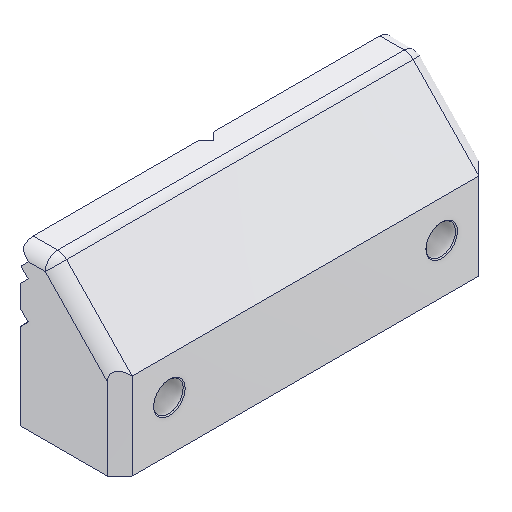
# Autodesk Inventor part: 3DP_ABS_Jaw_Second_Half
Saved by Autodesk Inventor 2026.1 (Build 301233000, 233)
## iProperties
Created: 2018-02-17
Part Number: 3DP_ABS_Jaw_Second_Half
Material: Ogólny
Document SubType Name: Modeling
Designer: Andrzej
Density: 1 g/cm^3
Appearance: PTFE
Mass: 38.2435 g
Surface Area: 91.1302 cm^2
Volume: 38.2435 cm^3
Author: Andrzej
Autodesk Inventor part; units mm, degrees
ref_plane "YZ Plane" through (0, 0, 0) normal (1, 0, 0) x (0, 1, 0)
ref_plane "XZ Plane" through (0, 0, 0) normal (0, 1, 0) x (-1, 0, 0)
sketch "Szkic1" plane through (0, 0, 0) normal (0, 0, 1) x (1, 0, 0)
  line L0 (-10, 37.5) -> (10, 37.5)
  line L1 (10, 37.5) -> (10, -37.5)
  line L2 (10, -37.5) -> (-10, -37.5)
  line L3 (-10, -37.5) -> (-10, 37.5)
  point P0 (0, 0)
  dimension "d0" = 20
  dimension "d1" = 75
  dimension "d39" = 37.5
  dimension "d40" = 10
  constraints: 8 end point, 2 parallel, 1 horizontal, 1 perpendicular
  measures "d0" distance of L1.end L2.end
  measures "d1" distance of L0.end L1.end
  measures "d39" distance from line of point (0, 0) L0
  measures "d40" distance from line of point (0, 0) L1
extrude "Wyciągnięcie proste1" add sketch "Szkic1" along normal blind 32
sketch "Szkic2" plane through (10, -37.5, 0) normal (1, 0, 0) x (0, 0, -1)
  line L0 (0, 75) -> (0, 0) projected
  line L1 (0, 75) -> (-32, 75) projected
  line L2 (-32, 0) -> (-32, 75) projected
  line L3 (0, 0) -> (-32, 0) projected
  point P0 (0, 37.5)
  point P1 (-10, 10)
  point P2 (-10, 65)
  dimension "d4" = 32
  dimension "d5" = 10
  dimension "d6" = 10
  dimension "d7" = 10
  dimension "d8" = 10
  measures "d4" distance of L0.end L2.start
  measures "d5" distance from line of L0 point (-10, 10)
  measures "d6" distance from line of L0 point (-10, 65)
  measures "d7" distance from line of L3 point (-10, 10)
  measures "d8" distance from line of L1 point (-10, 65)
hole "Otwór1" at (10, -27.5, 10) at (10, 27.5, 10) direction (-1, 0, 0) diameter 6 end through all
sketch "Szkic3" plane through (-10, 37.5, 0) normal (0, 1, 0) x (1, 0, 0)
  line L0 (0, 0) -> (20, 0) projected
  line L1 (0, 0) -> (0, -32) projected
  line L2 (20, -32) -> (0, -32) projected
  line L3 (20, 0) -> (20, -32) projected
  line L4 (0, -28) -> (1.5, -26.5)
  line L5 (0, -28) -> (2.2095, -28) construction
  line L6 (0, 0) -> (0, -32) projected
  line L7 (0, -25) -> (1.5, -26.5)
  line L8 (0, -25) -> (2.7592, -25) construction
  dimension "d17" = 45
  dimension "d19" = 45
  dimension "d20" = 3
  dimension "d21" = 4
  constraints: 8 end point, 2 horizontal, 2 point on line
  measures "d17" angle of L5 L4
  measures "d19" angle of L7 L8
  measures "d20" distance of L7.start L4.start
  measures "d21" distance from line of L2 L4.start
extrude "Wyciągnięcie proste2" cut sketch "Szkic3" against normal through all contours L7 L4 L1
chamfer "Faza1" distance 14 distance2 14.5 1 edges at (10, 0, 32) measured on face at (-3.3333, 12.5, 32)
chamfer "Faza2" distance 2.5 angle 45 2 edges at (10, -37.5, 8.75) (10, 37.5, 8.75)
ref_plane "Płaszczyzna konstrukcyjna1" through (-10, 37.5, 32) normal (0, -0.9902681, -0.1391731) x (-1, 0, 0)
sketch "Szkic4" plane through (-10, 37.5, 32) normal (0, -0.9902681, -0.1391731) x (-1, 0, 0)
  line L0 (-17.5, 31.6886) -> (-17.5, 11.7948) projected
  line L1 (0, 31.6886) -> (-17.5, 31.6886) projected
  line L2 (0, 31.6886) -> (0, 6.9319) projected
  line L3 (0, 6.9319) -> (-1.5, 5.4465) projected
  line L4 (-1.5, 5.4465) -> (0, 3.9611) projected
  line L5 (0, 3.9611) -> (0, 0) projected
  line L6 (-6, 0) -> (0, 0) projected
  line L7 (-17.5, 11.7948) -> (-6, 0) projected
  line L8 (0, -3.5061) -> (0, 6.9319) projected
  line L9 (0, 1) -> (-1.5, 2.5)
  line L10 (0, 1) -> (2.5951, 1) construction
  line L11 (0, 31.6886) -> (0, 6.9319) projected
  line L12 (0, 4) -> (-1.5, 2.5)
  line L13 (0, 4) -> (3.5979, 4) construction
  line L14 (0, 1) -> (0, 4)
  point P0 (-10, 26.4696)
  dimension "d32" = 135
  dimension "d34" = 135
  dimension "d35" = 3
  dimension "d36" = 1
  constraints: 10 end point, 2 horizontal, 2 point on line, 1 collinear
  measures "d32" angle of L10 L9
  measures "d34" angle of L12 L13
  measures "d35" distance of L12.start L9.start
  measures "d36" distance of L5.end L9.start
extrude "Wyciągnięcie proste3" cut sketch "Szkic4" along normal through all contours L8 L4 L12 | L9 L12 L4 L5
mirror "Odbicie lustrzane1" about plane through (0, 0, 0) normal (0, 1, 0) of "Wyciągnięcie proste3"
sketch "Szkic5" plane through (0, 0, 32) normal (0, 0, 1) x (1, 0, 0)
  line L0 (-4, 37.5) -> (-4, -37.5) projected
  line L1 (-4, 37.5) -> (-10, 37.5) projected
  line L2 (-10, 37.5) -> (-10, -37.5) projected
  line L3 (-10, -37.5) -> (-4, -37.5) projected
  line L4 (-10, 1.5) -> (-4.369, 1.5) construction
  line L5 (-10, -37.5) -> (-10, 0) projected
  line L6 (-10, -1.5) -> (-2.768, -1.5) construction
  line L7 (-10, -1.5) -> (-8.5, 0)
  line L8 (-10, 1.5) -> (-8.5, 0)
  point P0 (0, 0)
  dimension "d45" = 3
  dimension "d46" = 45
  dimension "d47" = 45
  dimension "d48" = 75
  dimension "d49" = 36
  constraints: 8 end point, 2 horizontal, 2 point on line, 1 perpendicular
  measures "d45" distance of L6.start L4.start
  measures "d46" angle of L4 L8
  measures "d47" angle of L6 L7
  measures "d48" distance of L1.end L2.end
  measures "d49" distance from line of L1 L4.start
extrude "Wyciągnięcie proste4" cut sketch "Szkic5" against normal through all contours L8 L7 L2
fillet "Zaokrąglenie1" radius 2.5 5 edges at (-4, 0, 32) (1.75, 37.5, 26.0446) (1.75, -37.5, 26.0446) (-7, -37.5, 32) (-7, 37.5, 32)
chamfer "Faza3" distance 0.2 angle 45 4 edges at (-10, 27.5, 13) (-10, -27.5, 13) (10, -27.5, 13) (10, 27.5, 13)
sketch "Szkic6" plane through (0, 0, 0) normal (0, 0, -1) x (-1, 0, 0)
  circle A0 centre (0, 0) radius 5
  line L0 (10, -1.5) -> (8.5, 0) projected
  line L1 (8.5, 0) -> (10, 1.5) projected
  line L2 (10, 1.5) -> (10, 37.5) projected
  line L3 (10, 37.5) -> (-7.5, 37.5) projected
  line L4 (-10, 35) -> (-7.5, 37.5) projected
  line L5 (-10, 35) -> (-10, -35) projected
  line L6 (-7.5, -37.5) -> (-10, -35) projected
  line L7 (-7.5, -37.5) -> (10, -37.5) projected
  line L8 (10, -37.5) -> (10, -1.5) projected
  point P0 (0, 0)
  dimension "d56" = 10
  dimension "d57" = 75
  dimension "d58" = 37.5
  dimension "d59" = 20
  dimension "d60" = 10
  constraints: 1 centre point
  measures "d56" diameter of A0
  measures "d57" distance between parallel lines of L7 L3
  measures "d58" distance from line of A0.centre L3
  measures "d59" distance between parallel lines of L2 L5
  measures "d60" distance from line of L5 A0.centre
extrude "Wyciągnięcie proste5" cut sketch "Szkic6" against normal blind 4.2 contours A0
chamfer "Faza4" distance 0.3 angle 45 1 edges at (5, 0, 0)
equation "\"d39\" = 0.5 * d1"
equation "\"d40\" = 0.5 * d0"
equation "\"d6\" = d5"
equation "\"d8\" = d7"
equation "\"d49\" = -0.5 * d45 + 0.5 * d48"
equation "\"d58\" = 0.5 * d57"
equation "\"d60\" = 0.5 * d59"
